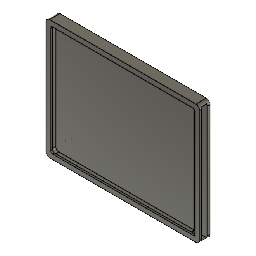
ipad_holder_2 v2 (Autodesk Fusion 360 design; units mm, degrees)
Autodesk Fusion 360 part; units mm, degrees
sketch "Sketch1" plane through (0, 0, 0) normal (0, 1, 0) x (1, 0, 0)
  line L0 (118.5, 97) -> (-118.5, 97)
  line L1 (-124.5, 91) -> (-124.5, -91)
  line L2 (-118.5, -97) -> (118.5, -97)
  line L3 (124.5, -91) -> (124.5, 91)
  line L4 (124.5, 97) -> (-124.5, -97) construction
  line L5 (-124.5, 97) -> (124.5, -97) construction
  arc A0 (118.5, -97) -> (124.5, -91) centre (118.5, -91) ccw
  arc A1 (-124.5, -91) -> (-118.5, -97) centre (-118.5, -91) ccw
  arc A2 (124.5, 91) -> (118.5, 97) centre (118.5, 91) ccw
  arc A3 (-118.5, 97) -> (-124.5, 91) centre (-118.5, 91) ccw
  dimension "d1" = 249
  dimension "d2" = 194
  dimension "d3" = 6
  dimension "d4" = 6
  dimension "d5" = 6
  dimension "d6" = 6
  constraint horizontal L0
  constraint perpendicular L0 L1
  constraint parallel L0 L2
  constraint parallel L1 L3
  constraint coincident L4 origin
  constraint coincident L5 origin
  constraint coincident L5.end L3
  constraint coincident L5.end L2
  constraint tangent L3 A0
  constraint tangent L2 A0
  constraint coincident L4.end L1
  constraint coincident L4.end L2
  constraint tangent L1 A1
  constraint tangent L2 A1
  constraint coincident L4.start L0
  constraint coincident L4.start L3
  constraint tangent L0 A2
  constraint tangent L3 A2
  constraint coincident L5.start L1
  constraint coincident L5.start L0
  constraint tangent L1 A3
  constraint tangent L0 A3
  measures "d1" distance of L4.end L5.end
  measures "d2" distance of L5.start L4.end
  measures "d3" radius of A0
  measures "d4" radius of A1
  measures "d5" radius of A2
  measures "d6" radius of A3
extrude "Extrude1" add sketch "Sketch1" along normal blind 17
sketch "Sketch2" plane through (0, 0, 0) normal (0, 1, 0) x (1, 0, 0)
  line L0 (115.75, 93.25) -> (-115.75, 93.25)
  line L1 (-120.75, 88.25) -> (-120.75, -88.25)
  line L2 (-115.75, -93.25) -> (115.75, -93.25)
  line L3 (120.75, -88.25) -> (120.75, 88.25)
  line L4 (120.75, 93.25) -> (-120.75, -93.25) construction
  line L5 (-120.75, 93.25) -> (120.75, -93.25) construction
  arc A0 (-120.75, -88.25) -> (-115.75, -93.25) centre (-115.75, -88.25) ccw
  arc A1 (115.75, -93.25) -> (120.75, -88.25) centre (115.75, -88.25) ccw
  arc A2 (-115.75, 93.25) -> (-120.75, 88.25) centre (-115.75, 88.25) ccw
  arc A3 (120.75, 88.25) -> (115.75, 93.25) centre (115.75, 88.25) ccw
  dimension "d9" = 241.5
  dimension "d10" = 186.5
  dimension "d11" = 5
  dimension "d12" = 5
  dimension "d13" = 5
  dimension "d14" = 5
  constraint horizontal L0
  constraint perpendicular L0 L1
  constraint parallel L0 L2
  constraint parallel L1 L3
  constraint coincident L4 origin
  constraint coincident L5 origin
  constraint coincident L4.end L2
  constraint coincident L4.end L1
  constraint tangent L2 A0
  constraint tangent L1 A0
  constraint coincident L5.end L2
  constraint coincident L5.end L3
  constraint tangent L2 A1
  constraint tangent L3 A1
  constraint coincident L5.start L1
  constraint coincident L5.start L0
  constraint tangent L1 A2
  constraint tangent L0 A2
  constraint coincident L4.start L3
  constraint coincident L4.start L0
  constraint tangent L3 A3
  constraint tangent L0 A3
  measures "d9" distance of L4.end L5.end
  measures "d10" distance of L5.start L4.end
  measures "d11" radius of A0
  measures "d12" radius of A1
  measures "d13" radius of A2
  measures "d14" radius of A3
ref_plane "WorkPlane1" through (0, 3, 0) normal (0, 1, 0) x (-1, 0, 0)
extrude "Extrude2" cut sketch "Sketch2" along normal blind 9.3
sketch "Sketch3" plane through (0, 0, 0) normal (0, -1, 0) x (1, 0, 0)
  line L0 (120.75, 88.25) -> (120.75, -88.25)
  arc A0 (115.75, -93.25) -> (120.75, -88.25) centre (115.75, -88.25) ccw
  line L1 (115.75, -93.25) -> (-115.75, -93.25)
  arc A1 (-120.75, -88.25) -> (-115.75, -93.25) centre (-115.75, -88.25) ccw
  line L2 (-120.75, -88.25) -> (-120.75, 88.25)
  arc A2 (-115.75, 93.25) -> (-120.75, 88.25) centre (-115.75, 88.25) ccw
  line L3 (-115.75, 93.25) -> (115.75, 93.25)
  arc A3 (120.75, 88.25) -> (115.75, 93.25) centre (115.75, 88.25) ccw
  arc A4 (-124.5, -91) -> (-118.5, -97) centre (-118.5, -91) ccw
  line L4 (-118.5, -97) -> (118.5, -97)
  arc A5 (118.5, -97) -> (124.5, -91) centre (118.5, -91) ccw
  line L5 (124.5, -91) -> (124.5, 91)
  arc A6 (124.5, 91) -> (118.5, 97) centre (118.5, 91) ccw
  line L6 (118.5, 97) -> (-118.5, 97)
  arc A7 (-118.5, 97) -> (-124.5, 91) centre (-118.5, 91) ccw
  line L7 (-124.5, 91) -> (-124.5, -91)
  line L8 (-113.5, 89) -> (113.5, 89)
  line L9 (116.5, 86) -> (116.5, -89)
  line L10 (116.5, -89) -> (-113.5, -89)
  line L11 (-116.5, -86) -> (-116.5, 86)
  line L12 (-116.5, 89) -> (116.5, -89) construction
  line L13 (116.5, 89) -> (-116.5, -89) construction
  arc A8 (-113.5, 89) -> (-116.5, 86) centre (-113.5, 86) ccw
  arc A9 (116.5, 86) -> (113.5, 89) centre (113.5, 86) ccw
  arc A10 (-116.5, -86) -> (-113.5, -89) centre (-113.5, -86) ccw
  dimension "d18" = 233
  dimension "d19" = 178
  dimension "d20" = 3
  dimension "d21" = 3
  dimension "d22" = 3
  constraint horizontal L8
  constraint perpendicular L8 L9
  constraint parallel L8 L10
  constraint parallel L9 L11
  constraint coincident L12 origin
  constraint coincident L13 origin
  constraint coincident L12.start L8
  constraint coincident L12.start L11
  constraint tangent L8 A8
  constraint tangent L11 A8
  constraint coincident L13.start L9
  constraint coincident L13.start L8
  constraint tangent L9 A9
  constraint tangent L8 A9
  constraint coincident L13.end L11
  constraint coincident L13.end L10
  constraint tangent L11 A10
  constraint tangent L10 A10
  measures "d18" distance of L9.end L13.end
  measures "d19" distance of L13.start L9.end
  measures "d20" radius of A8
  measures "d21" radius of A9
  measures "d22" radius of A10
sketch "Sketch4" plane through (124.5, 0, 0) normal (1, 0, 0) x (0, 1, 0)
  line L0 (0, 91) -> (0, -91)
  line L1 (0, -91) -> (17, -91)
  line L2 (17, -91) -> (17, 91)
  line L3 (17, 91) -> (0, 91)
  line L4 (3, 94) -> (12.2, 94)
  line L5 (12.2, 94) -> (12.2, -94)
  line L6 (12.2, -94) -> (3, -94)
  line L7 (3, -94) -> (3, 94)
  dimension "d23" = 9.2
  dimension "d24" = 188
  constraint horizontal L4
  constraint vertical L5
  constraint horizontal L6
  constraint vertical L7
  measures "d23" distance of L4.start L4.end
  measures "d24" distance of L4.start L6.end
extrude "Extrude3" cut sketch "Sketch4" against normal blind 6 contours L3 L4 L5 L7 | L1 L3 L5 L7 | L1 L5 L6 L7
sketch "Sketch5" plane through (0, 17, 0) normal (0, 1, 0) x (-1, 0, 0)
  arc A0 (118.5, -97) -> (124.5, -91) centre (118.5, -91) ccw
  line L0 (124.5, -91) -> (124.5, 91)
  arc A1 (124.5, 91) -> (118.5, 97) centre (118.5, 91) ccw
  line L1 (118.5, 97) -> (-118.5, 97)
  arc A2 (-118.5, 97) -> (-124.5, 91) centre (-118.5, 91) ccw
  line L2 (-124.5, 91) -> (-124.5, -91)
  arc A3 (-124.5, -91) -> (-118.5, -97) centre (-118.5, -91) ccw
  line L3 (-118.5, -97) -> (118.5, -97)
  circle A4 centre (-100, 70) radius 6
  circle A5 centre (100, 70) radius 6
  circle A6 centre (-100, -70) radius 6
  circle A7 centre (100, -70) radius 6
  dimension "d27" = 12
  dimension "d28" = 12
  dimension "d29" = 12
  dimension "d30" = 12
  measures "d27" diameter of A4
  measures "d28" diameter of A5
  measures "d29" diameter of A6
  measures "d30" diameter of A7
extrude "Extrude4" cut sketch "Sketch5" against normal blind 3.5 contours A4 | A5 | A6 | A7
extrude "Extrude5" add sketch "Sketch3" against normal blind 3 contours L0 A0 L1 A1 L2 A2 L3 A3
sketch "Sketch6" plane through (118.5, 0, 0) normal (1, 0, 0) x (0, 1, 0)
  line L0 (9.3, -92.4258) -> (3, -92.4258)
  line L1 (3, -92.4258) -> (3, -94)
  line L2 (3, -94) -> (12.2, -94)
  line L3 (12.2, -94) -> (12.2, 94)
  line L4 (12.2, 94) -> (3, 94)
  line L5 (3, 94) -> (3, 92.4258)
  line L6 (3, 92.4258) -> (9.3, 92.4258)
  line L7 (9.3, 92.4258) -> (9.3, -92.4258)
  line L8 (3, 94) -> (12.2, 94)
  line L9 (12.2, 94) -> (12.2, -94)
  line L10 (12.2, -94) -> (3, -94)
  line L11 (3, -94) -> (3, 94)
  constraint horizontal L8
  constraint vertical L9
  constraint horizontal L10
  constraint vertical L11
  constraint coincident L2.end L3.start
  constraint coincident L4.end L5.start
extrude "Extrude6" cut sketch "Sketch6" against normal blind 15
sketch "Sketch7" plane through (0, 3, 0) normal (0, 1, 0) x (1, 0, 0)
extrude "Extrude7" cut 1 faces at (-42.6667, 9.3, -31.0833) along direction (0, 1, 0) blind 3
